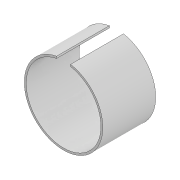
# Autodesk Inventor part: case
Saved by Autodesk Inventor 2020 (Build 240168000, 168)
## iProperties
Created: 2020-08-28
Part Number: case
Material: 일반
Document SubType Name: Modeling
Designer: 이호석
Mass: 4.24424 g
Surface Area: 80.669 cm^2
Volume: 4.24424 cm^3
Density: 1 g/cm^3
Appearance: 기본값
Author: 이호석
Autodesk Inventor part; units mm, degrees
ref_plane "YZ Plane" through (0, 0, 0) normal (1, 0, 0) x (0, 1, 0)
ref_plane "XZ Plane" through (0, 0, 0) normal (0, 1, 0) x (-1, 0, 0)
ref_plane "XY Plane" through (0, 0, 0) normal (0, 0, 1) x (1, 0, 0)
sketch "스케치1" plane through (0, 0, 0) normal (0, 0, 1) x (1, 0, 0)
  circle A0 centre (0, 0) radius 21.2
  circle A1 centre (0, 0) radius 22.3
  line L0 (0, 0) -> (-4, 0)
  line L1 (-4, 0) -> (4, 0)
  line L2 (4, 0) -> (4, 21.9383)
  line L3 (-4, 0) -> (-4, 21.9383)
  point P0 (-4, 20.8192)
  point P1 (4, 20.8192)
  dimension "d0" = 42.4
  dimension "d1" = 44.6
  dimension "d2" = 4
  dimension "d3" = 8
  constraints: 8 end point, 2 centre point, 2 coincident, 2 point on circle, 1 horizontal, 1 parallel, 1 perpendicular, 1 point on line
  measures "d0" diameter of A0
  measures "d1" diameter of A1
  measures "d2" distance of L0.start L0.end
  measures "d3" distance of L0.end L1.end
extrude "돌출1" add sketch "스케치1" along normal blind 30 contours A0 L2 A1 L3 picked at (21.5236, -3.4225)
